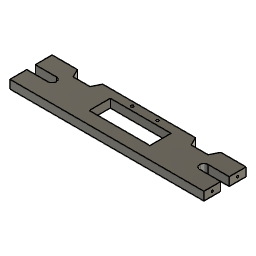
Querverstrebung_230mm_250606 (Autodesk Fusion 360 design; units mm, degrees)
Autodesk Fusion 360 part; units mm, degrees
sketch "Skizze1" plane through (0, 0, 0) normal (0, 0, 1) x (1, 0, 0)
  line L0 (0, 0) -> (230, 0)
  line L1 (230, 0) -> (230, 20)
  line L2 (230, 20) -> (205, 20)
  line L3 (230, 30) -> (205, 30)
  line L4 (230, 30) -> (230, 50)
  line L5 (230, 50) -> (200, 50)
  line L6 (170, 50) -> (175, 40)
  line L7 (175, 40) -> (195, 40)
  line L8 (200, 50) -> (195, 40)
  line L9 (55, 40) -> (35, 40)
  line L10 (55, 40) -> (60, 50)
  line L11 (35, 40) -> (30, 50)
  line L12 (30, 50) -> (0, 50)
  line L13 (0, 50) -> (0, 30)
  line L14 (0, 30) -> (25, 30)
  line L15 (0, 0) -> (0, 20)
  line L16 (0, 20) -> (25, 20)
  arc A0 (25, 20) -> (25, 30) centre (25, 25) ccw
  arc A1 (205, 30) -> (205, 20) centre (205, 25) ccw
  line L17 (115, 40) -> (79, 40)
  line L18 (115, 40) -> (151, 40)
  line L19 (79, 40) -> (79, 15)
  line L20 (79, 15) -> (151, 15)
  line L21 (151, 15) -> (151, 40)
  circle A2 centre (100, 45) radius 1.6
  circle A3 centre (130, 45) radius 1.6
  line L22 (60, 50) -> (170, 50)
  dimension "d1" = 230
  dimension "d2" = 20
  dimension "d3" = 25
  dimension "d6" = 10
  dimension "d7" = 25
  dimension "d8" = 20
  dimension "d9" = 30
  dimension "d11" = 30
  dimension "d14" = 20
  dimension "d15" = 110
  dimension "d18" = 20
  dimension "d20" = 30
  dimension "d21" = 20
  dimension "d22" = 25
  dimension "d23" = 20
  dimension "d24" = 25
  dimension "d27" = 36
  dimension "d28" = 36
  dimension "d29" = 25
  dimension "d30" = 72
  dimension "d33" = 3.2
  constraint coincident L0.start L15.start
  constraint horizontal L0
  constraint perpendicular L0 L1
  constraint perpendicular L1 L2
  constraint perpendicular L3 L4
  constraint perpendicular L4 L5
  constraint horizontal L7
  constraint horizontal L12
  constraint perpendicular L12 L13
  constraint perpendicular L13 L14
  constraint perpendicular L0 L15
  constraint perpendicular L15 L16
  constraint tangent L16 A0
  constraint tangent L2 A1
  constraint perpendicular L17 L19
  constraint perpendicular L19 L20
  constraint horizontal L22
  measures "d1" distance of L0.start L0.end
  measures "d2" distance of L0.end L1.end
  measures "d3" distance of L1.end L2.end
  measures "d6" distance of L1.end L3.start
  measures "d7" distance of L3.start L3.end
  measures "d8" distance of L3.start L4.end
  measures "d9" distance of L4.end L5.end
  measures "d11" distance of L5.end L6.start
  measures "d14" distance of L6.end L7.end
  measures "d15" distance of L6.start L10.end
  measures "d18" distance of L9.start L9.end
  measures "d20" distance of L11.end L12.end L10
  measures "d21" distance of L12.end L13.end
  measures "d22" distance of L13.end L14.end
  measures "d23" distance of L0.start L15.end
  measures "d24" distance of L15.end L16.end
  measures "d27" distance of L17.start L17.end
  measures "d28" distance of L17.start L18.end
  measures "d29" distance of L17.end L19.end
  measures "d30" distance of L19.end L20.end
  measures "d33" diameter of A2
extrude "Extrusion1" add sketch "Skizze1" along normal blind 10
sketch "Skizze2" plane through (230, 0, 0) normal (1, 0, 0) x (0, 1, 0)
  line L0 (0, 0) -> (20, 0)
  line L1 (20, 0) -> (20, 10)
  line L2 (20, 10) -> (0, 10)
  line L3 (0, 10) -> (0, 0)
  line L4 (0, 10) -> (20, 0)
  line L5 (20, 10) -> (0, 0)
  line L6 (49.9281, 0) -> (49.9281, 10)
  circle A0 centre (10, 5) radius 1.2
  dimension "d36" = 2.4
  constraint coincident L2.end L3.start
  constraint coincident L0.end L1.start
  constraint coincident L1.end L2.start
  constraint coincident L0.start L3.end
  constraint perpendicular L2 L6
  constraint midpoint L4 A0.centre
  measures "d36" diameter of A0
sketch "Skizze3" plane through (230, 0, 0) normal (1, 0, 0) x (0, 1, 0)
  line L0 (30, 0) -> (50, 0)
  line L1 (50, 0) -> (50, 10)
  line L2 (50, 10) -> (30, 10)
  line L3 (30, 10) -> (30, 0)
  line L4 (30, 10) -> (50, 0)
  line L5 (50, 10) -> (30, 0)
  circle A0 centre (40, 5) radius 1.2
  dimension "d37" = 2.4
  constraint coincident L2.end L3.start
  constraint coincident L0.end L1.start
  constraint coincident L1.end L2.start
  constraint coincident L0.start L3.end
  constraint midpoint L5 A0.centre
  measures "d37" diameter of A0
sketch "Skizze4" plane through (0, 0, 0) normal (-1, 0, 0) x (0, -1, 0)
  line L0 (-50, 0) -> (-30, 0)
  line L1 (-30, 0) -> (-30, 10)
  line L2 (-30, 10) -> (-50, 10)
  line L3 (-50, 10) -> (-50, 0)
  line L4 (-50, 10) -> (-30, 0)
  line L5 (-30, 10) -> (-50, 0)
  line L6 (0, 0) -> (0, 10)
  circle A0 centre (-40, 5) radius 1
  dimension "d38" = 2
  constraint coincident L2.end L3.start
  constraint coincident L0.end L1.start
  constraint coincident L1.end L2.start
  constraint coincident L0.start L3.end
  constraint coincident L6.start origin
  constraint parallel L1 L6
  constraint midpoint L4 A0.centre
  measures "d38" diameter of A0
sketch "Skizze5" plane through (0, 0, 0) normal (-1, 0, 0) x (0, -1, 0)
  line L0 (-20, 0) -> (0, 0)
  line L1 (0, 0) -> (0, 10)
  line L2 (0, 10) -> (-20, 10)
  line L3 (-20, 10) -> (-20, 0)
  line L4 (-20, 10) -> (0, 0)
  line L5 (0, 10) -> (-20, 0)
  circle A0 centre (-10, 5) radius 1
  dimension "d39" = 2
  constraint coincident L2.end L3.start
  constraint coincident L0.end L1.start
  constraint coincident L1.end L2.start
  constraint coincident L0.start L3.end
  constraint midpoint L4 A0.centre
  measures "d39" diameter of A0
hole "Bohrung1" at (230, 10, 5) direction (-1, 0, 0) diameter 2.4 depth 20 tip angle 118
hole "Bohrung2" at (230, 40, 5) direction (-1, 0, 0) diameter 2.4 depth 20 tip angle 118
hole "Bohrung3" at (0, 10, 5) direction (1, 0, 0) diameter 2.4 depth 20 tip angle 118
hole "Bohrung4" at (0, 40, 5) direction (1, 0, 0) diameter 2.4 depth 20 tip angle 118
equation "d36 = Montagelochdurchmesser"
equation "d37 = Montagelochdurchmesser"
equation "d41 = Montagelochdurchmesser"
equation "d44 = Montagelochdurchmesser"
equation "d47 = Montagelochdurchmesser"
equation "d50 = Montagelochdurchmesser"
equation "Montagelochdurchmesser = 2.4 mm"
